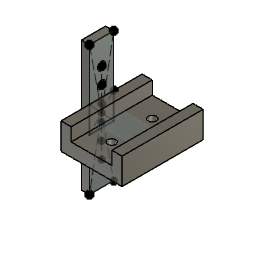
Slide Connector v2 (1) (Autodesk Fusion 360 design; units mm, degrees)
Autodesk Fusion 360 part; units mm, degrees
sketch "Sketch1" plane through (0, 0, 0) normal (0, 0, 1) x (1, 0, 0)
  line L0 (0, 0) -> (4, 0)
  line L1 (4, 0) -> (4, 12)
  line L2 (4, 12) -> (0, 12)
  line L3 (0, 12) -> (0, 0)
  dimension "d1" = 12
  dimension "d2" = 4
  constraint horizontal L0
  constraint vertical L1
  constraint horizontal L2
  constraint vertical L3
  constraint coincident L0.start L3.end
  measures "d1" distance of L0.start L2.end
  measures "d2" distance of L0.start L0.end
extrude "Extrude1" add sketch "Sketch1" along normal blind 64
sketch "Sketch2" plane through (4, 0, 0) normal (1, 0, 0) x (0, 1, 0)
  line L0 (0, 0) -> (12, 0)
  line L1 (12, 0) -> (12, 64)
  line L2 (12, 64) -> (0, 64)
  line L3 (0, 64) -> (0, 0)
  line L4 (0, 64) -> (12, 0) construction
  line L5 (12, 64) -> (0, 0) construction
  line L6 (12, 38.5) -> (0, 38.5)
  line L7 (0, 38.5) -> (0, 25.5)
  line L8 (0, 25.5) -> (12, 25.5)
  line L9 (12, 25.5) -> (12, 38.5)
  line L10 (12, 38.5) -> (0, 25.5) construction
  line L11 (0, 38.5) -> (12, 25.5) construction
  line L12 (6, 32) -> (6, 36) construction
  line L13 (6, 36) -> (6, 44) construction
  line L14 (6, 44) -> (6, 52) construction
  line L15 (6, 32) -> (6, 28) construction
  line L16 (6, 28) -> (6, 20) construction
  line L17 (6, 20) -> (6, 12) construction
  point P0 (6, 32)
  point P1 (6, 52)
  point P2 (6, 44)
  point P3 (6, 36)
  point P4 (6, 28)
  point P5 (6, 20)
  point P6 (6, 12)
  dimension "d5" = 13
  dimension "d6" = 4
  dimension "d7" = 8
  dimension "d8" = 8
  dimension "d9" = 4
  dimension "d10" = 8
  dimension "d11" = 8
  dimension "d20" = 12
  constraint coincident L2.end L3.start
  constraint coincident L0.end L1.start
  constraint coincident L1.end L2.start
  constraint coincident L0.start L3.end
  constraint horizontal L6
  constraint perpendicular L6 L7
  constraint parallel L6 L8
  constraint parallel L7 L9
  constraint coincident L10 P0
  constraint coincident L11 P0
  constraint coincident L1 L6.start
  constraint midpoint L4 P0
  constraint coincident P0 L12.start
  constraint perpendicular L6 L12
  constraint perpendicular L6 L13
  constraint parallel L13 L14
  constraint coincident P1 L14.end
  constraint coincident P2 L13.end
  constraint coincident P3 L12.end
  constraint perpendicular L8 L15
  constraint perpendicular L8 L16
  constraint parallel L16 L17
  constraint coincident P4 L15.end
  constraint coincident P5 L16.end
  constraint coincident P6 L17.end
  measures "d5" distance of L6.end L7.end
  measures "d6" distance of P0 P3
  measures "d7" distance of P3 P2
  measures "d8" distance of P2 P1
  measures "d9" distance of P0 P4
  measures "d10" distance of P4 P5
  measures "d11" distance of P5 P6
  measures "d20" distance of L6.start L6.end
extrude "Extrude2" add sketch "Sketch2" along normal blind 5 contours L1 L3 L6 L7 L8 L9
sketch "Sketch3" plane through (9, 0, 0) normal (1, 0, 0) x (0, 1, 0)
  line L0 (12, 25.5) -> (12, 38.5)
  line L1 (12, 38.5) -> (0, 38.5)
  line L2 (0, 38.5) -> (0, 25.5)
  line L3 (0, 25.5) -> (12, 25.5)
  line L4 (0, 25.5) -> (12, 25.5)
  line L5 (12, 25.5) -> (12, 32)
  line L6 (12, 32) -> (0, 32)
  line L7 (0, 32) -> (0, 25.5)
  constraint horizontal L4
  constraint vertical L5
  constraint horizontal L6
  constraint vertical L7
  constraint midpoint L0 L5.end
  constraint coincident L2.end L3.start
extrude "Extrude3" add sketch "Sketch3" along normal blind 20.11 contours L0 L2 L3 L4 L5 L6 L7
sketch "Sketch4" plane through (29.11, 0, 0) normal (1, 0, 0) x (0, 1, 0)
  line L0 (0, 32) -> (0, 25.5)
  line L1 (0, 25.5) -> (12, 25.5)
  line L2 (12, 25.5) -> (12, 32)
  line L3 (12, 32) -> (0, 32)
  line L4 (0, 25.5) -> (12, 25.5)
  line L5 (12, 25.5) -> (12, 38.5)
  line L6 (12, 38.5) -> (0, 38.5)
  line L7 (0, 38.5) -> (0, 25.5)
  dimension "d16" = 12
  dimension "d17" = 13
  constraint horizontal L4
  constraint vertical L5
  constraint horizontal L6
  constraint vertical L7
  constraint coincident L0.end L1.start
  measures "d16" distance of L0.end L1.end
  measures "d17" distance of L1.end L5.end
extrude "Extrude4" add sketch "Sketch4" along normal blind 5
sketch "Sketch5" plane through (0, 0, 32) normal (0, 0, 1) x (-1, 0, 0)
  line L0 (-9, -12) -> (-9, 0)
  line L1 (-9, 0) -> (-29.11, 0)
  line L2 (-29.11, 0) -> (-29.11, -12)
  line L3 (-29.11, -12) -> (-9, -12)
hole "Hole1" at (4, 6, 52) at (4, 6, 44) at (4, 6, 20) at (4, 6, 12) direction (-1, 0, 0) diameter 4 depth 15 tip angle 180
sketch "Sketch6" plane through (0, 12, 0) normal (0, 1, 0) x (-1, 0, 0)
  line L0 (-4, 0) -> (0, 0)
  line L1 (0, 0) -> (0, 64)
  line L2 (0, 64) -> (-4, 64)
  line L3 (-4, 64) -> (-4, 38.5)
  line L4 (-4, 38.5) -> (-9, 38.5)
  line L5 (-9, 38.5) -> (-9, 32)
  line L6 (-9, 32) -> (-29.11, 32)
  line L7 (-29.11, 32) -> (-29.11, 38.5)
  line L8 (-29.11, 38.5) -> (-34.11, 38.5)
  line L9 (-34.11, 38.5) -> (-34.11, 25.5)
  line L10 (-34.11, 25.5) -> (-4, 25.5)
  line L11 (-4, 25.5) -> (-4, 0)
  line L12 (-4, 38.5) -> (-4, 25.5)
  line L13 (-4, 38.5) -> (-9, 38.5)
  line L14 (-9, 38.5) -> (-9, 32)
  line L15 (-9, 32) -> (-29.11, 32)
  line L16 (-29.11, 38.5) -> (-29.11, 32)
  line L17 (-29.11, 38.5) -> (-34.11, 38.5)
  line L18 (-34.11, 25.5) -> (-34.11, 38.5)
  line L19 (-4, 25.5) -> (-34.11, 25.5)
  constraint coincident L3.end L4.start
  constraint coincident L10.end L11.start
  constraint coincident L4.end L5.start
  constraint coincident L5.end L6.start
  constraint coincident L6.end L7.start
  constraint coincident L7.end L8.start
  constraint coincident L8.end L9.start
  constraint coincident L9.end L10.start
extrude "Extrude5" add sketch "Sketch6" along normal blind 14 contours L4 L5 L6 L7 L8 L9 L10 L12 L13 L14 L15 L16 L17 L18 L19
sketch "Sketch7" plane through (0, 0, 0) normal (0, -1, 0) x (1, 0, 0)
  line L0 (0, 0) -> (4, 0)
  line L1 (4, 0) -> (4, 25.5)
  line L2 (4, 25.5) -> (34.11, 25.5)
  line L3 (34.11, 25.5) -> (34.11, 38.5)
  line L4 (34.11, 38.5) -> (29.11, 38.5)
  line L5 (29.11, 38.5) -> (29.11, 32)
  line L6 (29.11, 32) -> (9, 32)
  line L7 (9, 32) -> (9, 38.5)
  line L8 (9, 38.5) -> (4, 38.5)
  line L9 (4, 38.5) -> (4, 64)
  line L10 (4, 64) -> (0, 64)
  line L11 (0, 64) -> (0, 0)
  line L12 (4, 38.5) -> (4, 25.5)
  line L13 (4, 25.5) -> (34.11, 25.5)
  line L14 (34.11, 25.5) -> (34.11, 38.5)
  line L15 (34.11, 38.5) -> (29.11, 38.5)
  line L16 (29.11, 38.5) -> (29.11, 32)
  line L17 (29.11, 32) -> (9, 32)
  line L18 (9, 32) -> (9, 38.5)
  line L19 (9, 38.5) -> (4, 38.5)
  constraint coincident L8.end L9.start
  constraint coincident L1.end L2.start
  constraint coincident L2.end L3.start
  constraint coincident L3.end L4.start
  constraint coincident L4.end L5.start
  constraint coincident L5.end L6.start
  constraint coincident L6.end L7.start
  constraint coincident L7.end L8.start
extrude "Extrude6" add sketch "Sketch7" along normal blind 14 contours L2 L3 L4 L5 L6 L7 L8 L12 L13 L14 L15 L16 L17 L18 L19
sketch "Sketch8" plane through (0, 0, 32) normal (0, 0, 1) x (-1, 0, 0)
  line L0 (-9, -26) -> (-9, 14)
  line L1 (-9, 14) -> (-29.11, 14)
  line L2 (-29.11, 14) -> (-29.11, -26)
  line L3 (-29.11, -26) -> (-9, -26)
  line L4 (-9, -26) -> (-29.11, 14) construction
  line L5 (-29.11, -26) -> (-9, 14) construction
  line L6 (-19.055, -6) -> (-19.055, -16) construction
  line L7 (-19.055, -6) -> (-19.055, 4)
  dimension "d28" = 10
  dimension "d29" = 10
  constraint coincident L0.start L3.end
  constraint coincident L1.end L2.start
  constraint coincident L2.end L3.start
  constraint coincident L0.end L1.start
  constraint midpoint L5 L6.start
  constraint perpendicular L3 L6
  constraint parallel L2 L7
  measures "d28" distance of L6.start L6.end
  measures "d29" distance of L6.start L7.end
hole "Hole2" at (19.055, -4, 32) at (19.055, 16, 32) direction (0, 0, -1) diameter 4 depth 50 tip angle 180
